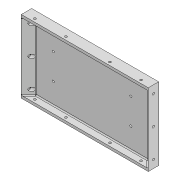
# Autodesk Inventor part: Print_Parts_V
Saved by Autodesk Inventor 2020 (Build 240168000, 168)
## iProperties
Created: 2021-02-11
Part Number: Print_Parts_V
Material: 一般
Document SubType Name: Modeling
Designer: ken113
Density: 1 g/cm^3
Appearance: 既定
Author: ken113
Autodesk Inventor part; units mm, degrees
ref_plane "YZ Plane" through (0, 0, 0) normal (1, 0, 0) x (0, 1, 0)
sketch "スケッチ1" plane through (0, 0, 0) normal (0, 0, 1) x (1, 0, 0)
  line L0 (122.5, -70) -> (-122.5, -70)
  line L1 (-122.5, -70) -> (-122.5, 70)
  line L2 (-122.5, 70) -> (122.5, 70)
  line L3 (122.5, 70) -> (122.5, -70)
  line L4 (122.5, -70) -> (-122.5, 70) construction
  line L5 (-122.5, -70) -> (122.5, 70) construction
  point P0 (0, 0)
  dimension "d0" = 245
  dimension "d1" = 140
  constraints: 12 end point, 2 midpoint, 2 parallel, 1 horizontal, 1 perpendicular
  measures "d0" distance of L1.end L2.end
  measures "d1" distance of L2.end L0.start
extrude "押し出し1" add sketch "スケッチ1" along normal blind 6
sketch "スケッチ2" plane through (0, 0, 6) normal (0, 0, 1) x (1, 0, 0)
  line L0 (-122.5, -70) -> (122.5, -70) projected
  line L1 (122.5, -70) -> (122.5, 70) projected
  line L2 (122.5, 70) -> (-122.5, 70) projected
  line L3 (-122.5, 70) -> (-122.5, -70) projected
  line L4 (-122.5, -70) -> (122.5, -70) projected
  line L5 (-122.5, 70) -> (-117.5, 70)
  line L6 (-117.5, 70) -> (-117.5, -70)
  line L7 (-117.5, -70) -> (-122.5, -70)
  line L8 (-122.5, -70) -> (-122.5, 70)
  line L9 (122.5, -70) -> (117.5, -70)
  line L10 (117.5, -70) -> (117.5, 70)
  line L11 (117.5, 70) -> (122.5, 70)
  line L12 (122.5, 70) -> (122.5, -70)
  point P0 (0, 0)
  dimension "d4" = 5
  dimension "d5" = 5
  constraints: 16 end point, 4 parallel, 2 horizontal, 2 perpendicular, 2 point on line
  measures "d4" distance between parallel lines of L6 L3
  measures "d5" distance between parallel lines of L1 L10
extrude "押し出し2" add sketch "スケッチ2" along normal blind 14 contours L3 L2 L6 L0 | L10 L2 L1 L0
sketch "スケッチ3" plane through (-122.5, -70, 0) normal (0, -1, 0) x (1, 0, 0)
  line L0 (0, 0) -> (245, 0) projected
  line L1 (245, 0) -> (245, 20) projected
  line L2 (240, 20) -> (245, 20) projected
  line L3 (240, 6) -> (240, 20) projected
  line L4 (5, 6) -> (240, 6) projected
  line L5 (5, 6) -> (5, 20) projected
  line L6 (0, 20) -> (5, 20) projected
  line L7 (0, 0) -> (0, 20) projected
  line L8 (0, 20) -> (5, 20) projected
  line L9 (0, 20) -> (14, 6)
  line L10 (240, 6) -> (5, 6) projected
  line L11 (245, 0) -> (245, 20) projected
  line L12 (245, 20) -> (231, 6)
  point P0 (122.5, 0)
  point P1 (240, 15)
  point P2 (5, 15)
  dimension "d14" = 45
  dimension "d15" = 45
  constraints: 4 end point, 2 point on line
  measures "d14" angle of L9 L4
  measures "d15" angle of L12 L4
extrude "押し出し3" add sketch "スケッチ3" against normal up to surface (140 mm away) contours L9 L4 L5 | L3 L4 L12
sketch "スケッチ5" plane through (-122.5, 70, 0) normal (0, 1, 0) x (1, 0, 0)
  line L0 (245, 0) -> (0, 0) projected
  line L1 (0, 0) -> (0, -20) projected
  line L2 (5, -20) -> (0, -20) projected
  line L3 (5, -15) -> (5, -20) projected
  line L4 (14, -6) -> (5, -15) projected
  line L5 (231, -6) -> (14, -6) projected
  line L6 (240, -15) -> (231, -6) projected
  line L7 (240, -15) -> (240, -20) projected
  line L8 (245, -20) -> (240, -20) projected
  line L9 (245, 0) -> (245, -20) projected
  line L10 (240, -15) -> (231, -6) projected
  line L11 (240, -15) -> (245, -20)
  line L12 (14, -6) -> (5, -15) projected
  line L13 (5, -15) -> (0, -20)
  point P0 (122.5, 0)
  constraints: 4 end point, 2 collinear
extrude "押し出し5" cut sketch "スケッチ5" against normal up to surface (140 mm away) contours L8 L7 L11 | L13 L3 L2
sketch "スケッチ6" plane through (122.5, -70, 0) normal (1, 0, 0) x (0, 0, -1)
  line L0 (0, 0) -> (0, 140) projected
  line L1 (0, 140) -> (-20, 140) projected
  line L2 (-20, 0) -> (-20, 140) projected
  line L3 (0, 0) -> (-20, 0) projected
  point P0 (0, 70)
  point P1 (-10, 15)
  point P2 (-10, 125)
  point P3 (-10, 70)
  dimension "d22" = 10
  dimension "d23" = 15
  dimension "d24" = 15
  dimension "d25" = 55
  constraints: 1 vertical alignment
  measures "d22" distance from line of point (-10, 15) L2
  measures "d23" distance from line of point (-10, 15) L3
  measures "d24" distance from line of L1 point (-10, 125)
  measures "d25" distance of point (-10, 70) point (-10, 15)
hole "穴1" at (122.5, -55, 10) at (122.5, 55, 10) at (122.5, 0, 10) direction (-1, 0, 0) diameter 4.3 end through all
ref_plane "作業平面1" through (108.5, -70, 0) normal (1, 0, 0) x (0, 0, -1)
sketch "スケッチ7" plane through (108.5, -70, 0) normal (1, 0, 0) x (0, 0, -1)
  circle A0 centre (-10, 125) radius 2.15 projected
  circle A1 centre (-10, 15) radius 2.15 projected
  circle A2 centre (-10, 70) radius 2.15 projected
  line L0 (-6, 140) -> (-20, 140) projected
  line L1 (-6, 0) -> (-6, 140) projected
  line L2 (-20, 0) -> (-6, 0) projected
  line L3 (-20, 0) -> (-20, 140) projected
  point P0 (0, 70)
hole "穴2" at (108.5, 55, 10) at (108.5, 0, 10) at (108.5, -55, 10) direction (1, 0, 0) diameter 7.5 depth 9
ref_plane "作業平面2" through (-108.5, -70, 0) normal (-1, 0, 0) x (0, 0, 1)
sketch "スケッチ8" plane through (-108.5, -70, 0) normal (-1, 0, 0) x (0, 0, 1)
  circle A0 centre (10, 125) radius 2.15 projected
  circle A1 centre (10, 15) radius 2.15 projected
  circle A2 centre (10, 70) radius 2.15 projected
  line L0 (20, 140) -> (6, 140) projected
  line L1 (20, 140) -> (20, 0) projected
  line L2 (6, 0) -> (20, 0) projected
  line L3 (6, 140) -> (6, 0) projected
  point P0 (0, 70)
hole "穴3" at (-108.5, -55, 10) at (-108.5, 0, 10) at (-108.5, 55, 10) direction (-1, 0, 0) diameter 7.5 depth 9
sketch "スケッチ9" plane through (-122.5, 70, 0) normal (0, 1, 0) x (1, 0, 0)
  line L0 (0, -20) -> (14, -6) projected
  line L1 (231, -6) -> (14, -6) projected
  line L2 (231, -6) -> (245, -20) projected
  line L3 (245, 0) -> (245, -20) projected
  line L4 (245, 0) -> (0, 0) projected
  line L5 (0, 0) -> (0, -20) projected
  line L6 (231, -6) -> (245, -20) projected
  line L7 (0, -20) -> (14, -6) projected
  line L8 (245, -20) -> (0, -20)
  point P0 (122.5, 0)
  constraints: 2 end point, 1 horizontal
extrude "押し出し6" add sketch "スケッチ9" against normal blind 5 contours L0 L1 L2 L8
sketch "スケッチ10" plane through (-122.5, -70, 0) normal (0, -1, 0) x (1, 0, 0)
  line L0 (245, 20) -> (231, 6) projected
  line L1 (245, 20) -> (0, 20) projected
  line L2 (14, 6) -> (0, 20) projected
  line L3 (231, 6) -> (14, 6) projected
  point P0 (122.5, 0)
extrude "押し出し7" add sketch "スケッチ10" against normal blind 5
sketch "スケッチ11" plane through (0, 0, 6) normal (0, 0, 1) x (1, 0, 0)
  line L0 (75, -25) -> (-75, -25)
  line L1 (-75, -25) -> (-75, 25)
  line L2 (-75, 25) -> (75, 25)
  line L3 (75, 25) -> (75, -25)
  line L4 (75, -25) -> (-75, 25) construction
  line L5 (-75, -25) -> (75, 25) construction
  point P0 (0, 0)
  point P1 (0, 0)
  point P2 (0, 0)
  point P3 (0, 0)
  dimension "d54" = 150
  dimension "d55" = 50
  constraints: 12 end point, 4 midpoint, 2 coincident, 2 parallel, 1 horizontal, 1 perpendicular
  measures "d54" distance of L1.end L2.end
  measures "d55" distance of L0.end L1.end
hole "穴4" at (-75, -25, 6) at (-75, 25, 6) at (75, -25, 6) at (75, 25, 6) direction (0, 0, -1) diameter 4.3 depth 9
sketch "スケッチ13" plane through (0, 0, 0) normal (0, 0, -1) x (-1, 0, 0)
  circle A0 centre (-75, -25) radius 2.15 projected
  circle A1 centre (75, -25) radius 2.15 projected
  circle A2 centre (75, 25) radius 2.15 projected
  circle A3 centre (-75, 25) radius 2.15 projected
  line L0 (122.5, -70) -> (-122.5, -70) projected
  line L1 (122.5, 70) -> (122.5, -70) projected
  line L2 (-122.5, 70) -> (122.5, 70) projected
  line L3 (-122.5, -70) -> (-122.5, 70) projected
  point P0 (0, 0)
hole "穴6" at (-75, 25, 0) at (-75, -25, 0) at (75, 25, 0) at (75, -25, 0) direction (0, 0, 1) diameter 4.3 depth 3 countersink diameter 8 countersink angle 90
fillet "フィレット1" radius 2 8 edges at (115.5, 65, 13) (0, 65, 6) (108.5, 0, 6) (115.5, -65, 13) (0, -65, 6) (-115.5, -65, 13) (-108.5, 0, 6) (-115.5, 65, 13)
sketch "スケッチ14" plane through (-122.5, 65, 0) normal (0, -1, 0) x (1, 0, 0)
  line L0 (242.1716, 20) -> (230.1716, 8) projected
  line L1 (242.1716, 20) -> (2.8284, 20) projected
  line L2 (14.8284, 8) -> (2.8284, 20) projected
  line L3 (230.1716, 8) -> (14.8284, 8) projected
  point P0 (122.5, 0)
  point P1 (20, 14)
  point P2 (225, 14)
  point P3 (165, 14)
  point P4 (80, 14)
  point P5 (0, 20)
  point P6 (245, 20)
  dimension "d78" = 6
  dimension "d79" = 20
  dimension "d80" = 20
  dimension "d81" = 60
  dimension "d82" = 60
  constraints: 3 horizontal alignment
  measures "d78" distance from line of L1 point (80, 14)
  measures "d79" horizontal distance of point (20, 14) point (0, 20)
  measures "d80" horizontal distance of point (245, 20) point (225, 14)
  measures "d81" distance of point (80, 14) point (20, 14)
  measures "d82" distance of point (225, 14) point (165, 14)
hole "穴7" at (-102.5, 65, 14) at (102.5, 65, 14) at (42.5, 65, 14) at (-42.5, 65, 14) direction (0, 1, 0) diameter 4.4 depth 9
sketch "スケッチ15" plane through (-122.5, 70, 0) normal (0, 1, 0) x (1, 0, 0)
  circle A0 centre (165, -14) radius 2.2 projected
  circle A1 centre (20, -14) radius 2.2 projected
  circle A2 centre (225, -14) radius 2.2 projected
  circle A3 centre (80, -14) radius 2.2 projected
  line L0 (245, 0) -> (245, -20) projected
  line L1 (245, 0) -> (0, 0) projected
  line L2 (0, 0) -> (0, -20) projected
  line L3 (0, -20) -> (245, -20) projected
  point P0 (122.5, 0)
hole "穴8" at (102.5, 70, 14) at (42.5, 70, 14) at (-42.5, 70, 14) at (-102.5, 70, 14) direction (0, -1, 0) diameter 4.4 end through all
